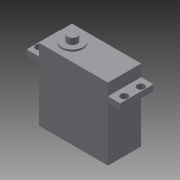
# Autodesk Inventor part: savox
Saved by Autodesk Inventor 2015 (Build 190159000, 159)
## iProperties
Created: 2015-06-27
Part Number: savox
Material: Genérico
Document SubType Name: Modeling
Designer: Roberto
Density: 1 g/cm^3
Appearance: Valor por defecto
Author: Roberto
Autodesk Inventor part; units mm, degrees
ref_plane "YZ Plane" through (0, 0, 0) normal (1, 0, 0) x (0, 1, 0)
ref_plane "XZ Plane" through (0, 0, 0) normal (0, 1, 0) x (-1, 0, 0)
ref_plane "XY Plane" through (0, 0, 0) normal (0, 0, 1) x (1, 0, 0)
sketch "Boceto1" plane through (0, 0, 0) normal (0, 1, 0) x (-1, 0, 0)
  line L0 (0, 0) -> (-40.9, 0)
  line L1 (-40.9, 0) -> (-40.9, -32)
  line L2 (-40.9, -32) -> (0, -32)
  line L3 (0, -32) -> (0, 0)
  dimension "d0" = 40.9
  dimension "d1" = 32
  constraints: 8 end point, 2 parallel, 1 horizontal, 1 perpendicular
  measures "d0" distance of L1.end L2.end
  measures "d1" distance of L0.end L1.end
extrude "Extrusión1" add sketch "Boceto1" along normal blind 19.6
sketch "Boceto2" plane through (0, 0, 0) normal (0, 0, 1) x (1, 0, 0)
  line L0 (20.45, 29.4794) -> (20.45, -8.3561)
  line L1 (0, 0) -> (0, 19.6) projected
  line L2 (0, 0) -> (0, 19.6) projected
  line L3 (20.45, 19.6) -> (-7.25, 19.6)
  line L4 (-7.25, 19.6) -> (-7.25, 0)
  line L5 (-7.25, 0) -> (20.45, 0)
  line L6 (0, 19.6) -> (40.9, 19.6) projected
  line L7 (0, 0) -> (40.9, 0) projected
  line L8 (-4.75, 38.1258) -> (-4.75, -18.5214)
  line L9 (50.1495, 9.8) -> (-24.2217, 9.8)
  circle A0 centre (-4.75, 14.7) radius 2.2
  circle A1 centre (-4.75, 4.9) radius 2.2
  line L10 (20.45, 0) -> (0, 0)
  line L11 (40.9, 19.6) -> (0, 19.6)
  line L12 (20.45, 0) -> (40.9, 0)
  line L13 (20.45, 19.6) -> (48.15, 19.6)
  line L14 (48.15, 19.6) -> (48.15, 0)
  line L15 (48.15, 0) -> (20.45, 0)
  circle A2 centre (45.65, 14.7) radius 2.2
  circle A3 centre (45.65, 4.9) radius 2.2
  dimension "d9" = 19.6
  dimension "d10" = 4.4
  dimension "d11" = 9.8
  dimension "d13" = 55.4
  dimension "d14" = 40.9
  dimension "d16" = 25.2
  constraints: 24 end point, 7 symmetric about line, 4 centre point, 3 collinear, 3 point on line, 2 horizontal, 2 midpoint, 2 parallel, 2 vertical, 1 equal radius, 1 perpendicular, 3 other
  measures "d9" diameter of L7 L9
  measures "d10" diameter of A1
  measures "d11" distance of A1.centre A0.centre
  measures "d13" diameter of L4 L0
  measures "d14" diameter of L1 L0
  measures "d16" distance between parallel lines of L0 L8
extrude "Extrusión2" add sketch "Boceto2" along normal blind 3.5 contours L6 L13 L14 L9 L0 | L0 L9 L1 L3 | L9 L14 L15 L7 L0 | L0 L5 L1 L9 | L1 L9 L8 A0 L3 | L1 L5 L8 A1 L9 | L8 A0 L9 L4 L3 | L8 A1 L5 L4 L9
sketch "Boceto3" plane through (0, 0, 3.5) normal (0, 0, 1) x (1, 0, 0)
  line L0 (0, 0) -> (40.9, 0)
  line L1 (40.9, 0) -> (40.9, 19.6)
  line L2 (40.9, 19.6) -> (0, 19.6)
  line L3 (0, 19.6) -> (0, 0)
  constraints: 8 end point, 2 parallel, 1 horizontal, 1 perpendicular
extrude "Extrusión3" add sketch "Boceto3" along normal blind 7
sketch "Boceto4" plane through (0, 0, 10.5) normal (0, 0, 1) x (1, 0, 0)
  circle A0 centre (10, 9.8) radius 6.3
  line L0 (0, 0) -> (40.9, 0) projected
  line L1 (0, 19.6) -> (0, 0) projected
  dimension "d21" = 12.6
  dimension "d22" = 9.8
  dimension "d23" = 10
  constraints: 1 centre point
  measures "d21" diameter of A0
  measures "d22" distance from line of L0 A0.centre
  measures "d23" distance from line of L1 A0.centre
extrude "Extrusión4" add sketch "Boceto4" along normal blind 1
sketch "Boceto5" plane through (10, 9.8, 11.5) normal (0, 0, 1) x (1, 0, 0)
  circle A0 centre (0, 0) radius 3
  circle A1 centre (0, 0) radius 6.3 projected
  point P0 (-10, -9.8)
  dimension "d26" = 6
  constraints: 1 centre point, 1 concentric
  measures "d26" diameter of A0
extrude "Extrusión5" add sketch "Boceto5" along normal blind 3.7 contours A0
sketch "Boceto6" plane through (0, 0, -32) normal (-1, 0, 0) x (0, 0, 1)
  line L0 (0, 0) -> (0, 19.6) projected
  line L1 (0, 13.3) -> (4.6057, 13.3)
  line L2 (4.6057, 13.3) -> (4.6057, 6.3)
  line L3 (4.6057, 6.3) -> (0, 6.3)
  line L4 (0, 6.3) -> (0, 13.3)
  line L5 (0, 19.6) -> (32, 19.6) projected
  line L6 (0, 0) -> (32, 0) projected
  dimension "d29" = 7
  dimension "d30" = 6.3
  dimension "d31" = 6.3
  constraints: 8 end point, 2 parallel, 1 horizontal, 1 perpendicular, 1 point on line
  measures "d29" distance of L1.end L2.end
  measures "d30" distance between parallel lines of L5 L1
  measures "d31" distance between parallel lines of L6 L3
extrude "Extrusión6" add sketch "Boceto6" along normal blind 6
